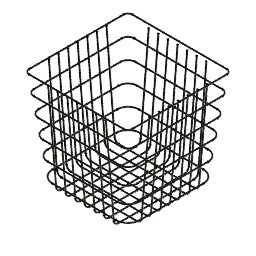
Living Roof Little Library Fusion Design File (Autodesk Fusion 360 archive; units mm, degrees)
design "Wire Basket"
Autodesk Fusion 360 part; units mm, degrees
note: some values were not read from the file. Chosen so that the rebuilt part matches the saved one: which bodies a step acts on.
sketch "Sketch1" plane through (0, 0, 0) normal (0, 1, 0) x (1, 0, 0)
  line L0 (0, 0) -> (104.7294, 0)
  line L1 (117.381, -11.5931) -> (139.7, -266.7)
  line L2 (0, -1.75) -> (0, -22.5)
  line L3 (1.75, 0) -> (22.5, 0)
  arc A0 (117.381, -11.5931) -> (104.7294, 0) centre (104.7294, -12.7) ccw
  line L4 (139.7, -266.7) -> (147.5, -266.7) construction
  circle A1 centre (143.7, -266.7) radius 2
  circle A2 centre (139.2902, -216.2955) radius 2
  circle A3 centre (134.8804, -165.891) radius 2
  circle A4 centre (130.4705, -115.4865) radius 2
  circle A5 centre (126.0607, -65.082) radius 2
  circle A6 centre (121.6509, -14.6776) radius 2
  dimension "d1" = 139.7
  dimension "d9" = 266.7
  dimension "d10" = 85
  dimension "d11" = 12.7
  dimension "d14" = 4
  dimension "d15" = 4
  dimension "d19" = 0
  constraint coincident L0.start origin
  constraint horizontal L0
  constraint tangent L0 A0
  constraint tangent L1 A0
  constraint horizontal L4
  constraint coincident L4 A1.centre
  measures "d1" distance of L1.end L2
  measures "d9" vertical distance of L0.start L1.end
  measures "d10" angle of L1 L3
  measures "d11" radius of A0
  measures "d14" diameter of A1
  measures "d15" distance of L1.end A1.centre
sketch "Sketch2" plane through (0, 0, 0) normal (1, 0, 0) x (0, 1, 0)
  circle A0 centre (0, 0) radius 2
  dimension "d12" = 4
  constraint coincident A0.centre origin
  measures "d12" diameter of A0
ref_plane "WorkPlane1" through (0, 0, 266.7) normal (0, 0, 1) x (1, 0, 0)
sweep "Sweep1" add profiles "Sketch2" path "Sketch1" along L0 A0 L1 section 1 makes body 1
sketch "Sketch3" plane through (0, 0, 266.7) normal (0, 0, 1) x (1, 0, 0)
  line L0 (0, 0) -> (0, -193.7) construction
  line L1 (143.7, 0) -> (143.7, -131)
  line L2 (131, -143.7) -> (0, -143.7)
  line L3 (0, 0) -> (143.7, -143.7) construction
  line L4 (135.0176, 0) -> (135.0176, -122.3176)
  line L5 (122.3176, -135.0176) -> (0, -135.0176)
  line L6 (126.3352, 0) -> (126.3352, -113.6352)
  line L7 (113.6352, -126.3352) -> (0, -126.3352)
  line L8 (117.6528, 0) -> (117.6528, -104.9528)
  line L9 (104.9528, -117.6528) -> (0, -117.6528)
  line L10 (108.9704, 0) -> (108.9704, -96.2704)
  line L11 (96.2704, -108.9704) -> (0, -108.9704)
  line L12 (100.288, 0) -> (100.288, -87.588)
  line L13 (87.588, -100.288) -> (0, -100.288)
  arc A0 (87.588, -100.288) -> (100.288, -87.588) centre (87.588, -87.588) ccw
  arc A1 (96.2704, -108.9704) -> (108.9704, -96.2704) centre (96.2704, -96.2704) ccw
  arc A2 (104.9528, -117.6528) -> (117.6528, -104.9528) centre (104.9528, -104.9528) ccw
  arc A3 (113.6352, -126.3352) -> (126.3352, -113.6352) centre (113.6352, -113.6352) ccw
  arc A4 (122.3176, -135.0176) -> (135.0176, -122.3176) centre (122.3176, -122.3176) ccw
  line L14 (0, 0) -> (147.5, 0) construction
  arc A5 (131, -143.7) -> (143.7, -131) centre (131, -131) ccw
  point P0 (143.7, 0)
  point P1 (139.2902, 0)
  point P2 (147.5, 0)
  dimension "d32" = 143.7
  dimension "d85" = 12.7
  dimension "d86" = 12.7
  dimension "d87" = 12.7
  dimension "d88" = 12.7
  dimension "d89" = 12.7
  dimension "d90" = 8.6824
  dimension "d91" = 8.6824
  dimension "d92" = 8.6824
  dimension "d93" = 8.6824
  dimension "d94" = 8.6824
  dimension "d95" = 12.7
  constraint coincident L0.start L3.start
  constraint vertical L0
  constraint coincident P0 L1.start
  constraint coincident L0 L2.end
  constraint perpendicular L0 L2
  constraint vertical L1
  constraint tangent L13 A0
  constraint tangent L12 A0
  constraint tangent L11 A1
  constraint tangent L10 A1
  constraint tangent L9 A2
  constraint tangent L8 A2
  constraint tangent L7 A3
  constraint tangent L6 A3
  constraint tangent L5 A4
  constraint tangent L4 A4
  constraint vertical L12
  constraint vertical L10
  constraint vertical L8
  constraint vertical L6
  constraint vertical L4
  constraint horizontal L5
  constraint horizontal L7
  constraint horizontal L9
  constraint horizontal L11
  constraint horizontal L13
  constraint coincident L3 A0.centre
  constraint coincident L3 A1.centre
  constraint coincident L3 A2.centre
  constraint coincident L3 A3.centre
  constraint coincident L3 A4.centre
  constraint coincident L0 L13.end
  constraint coincident L0 L11.end
  constraint coincident L0 L9.end
  constraint coincident L0 L7.end
  constraint coincident L0 L5.end
  constraint coincident P2 L14.end
  constraint coincident L14 L12.start
  constraint coincident L14 L10.start
  constraint coincident L14 L8.start
  constraint coincident L14 L6.start
  constraint coincident L14 L4.start
  constraint coincident L2 L3.end
  constraint coincident L1 L3.end
  constraint tangent L2 A5
  constraint tangent L1 A5
  measures "d32" distance of L0.start L2
  measures "d85" radius of A0
  measures "d86" radius of A1
  measures "d87" radius of A2
  measures "d88" radius of A3
  measures "d89" radius of A4
  measures "d90" distance of L2 L5
  measures "d91" distance of L5 L7
  measures "d92" distance of L7 L9
  measures "d93" distance of L9 L11
  measures "d94" distance of L11 L13
  measures "d95" radius of A5
sweep "Sweep2" add profiles "Sketch1" path "Sketch3" along L2 A5 L1 section 1 contours A1 separate body makes body 2
sweep "Sweep3" add profiles "Sketch1" path "Sketch3" along L12 A0 L13 section 1 contours A6 separate body makes body 3
sweep "Sweep4" add profiles "Sketch1" path "Sketch3" along L11 A1 L10 section 1 contours A5 separate body makes body 4
sweep "Sweep5" add profiles "Sketch1" path "Sketch3" along L9 A2 L8 section 1 contours A4 separate body makes body 5
sweep "Sweep6" add profiles "Sketch1" path "Sketch3" along L6 A3 L7 section 1 contours A3 separate body makes body 6
sweep "Sweep7" add profiles "Sketch1" path "Sketch3" along L5 A4 L4 section 1 contours A2 separate body makes body 7
pattern_linear "R-Pattern1" count 4 spacing 26.6667 along (0, -1, 0) of bodies 1 makes body 8 at (131.8461, -28.623, 181.7006) makes body 9 at (131.8461, -55.2896, 181.7006) makes body 10 at (131.8461, -81.9563, 181.7006)
mirror "Mirror1" about plane through (0, 0, 0) normal (1, 0, 0) of bodies 1 8 9 10 makes body 11 at (-131.8461, -1.9563, 181.7006) makes body 12 at (-131.8461, -28.623, 181.7006) makes body 13 at (-131.8461, -55.2896, 181.7006) makes body 14 at (-131.8461, -81.9563, 181.7006)
mirror "Mirror2" about plane through (0, 0, 0) normal (0, 1, 0) of bodies 14 12 13 8 9 10 makes body 15 at (131.8461, 28.623, 181.7006) makes body 16 at (131.8461, 55.2896, 181.7006) makes body 17 at (131.8461, 81.9563, 181.7006) makes body 18 at (-131.8461, 28.623, 181.7006) makes body 19 at (-131.8461, 55.2896, 181.7006) makes body 20 at (-131.8461, 81.9563, 181.7006)
mirror "Mirror3" about plane through (0, 0, 0) normal (1, 0, 0) of bodies 2 4 3 6 5 7 makes body 21 at (-145.6382, -43.6667, 267.1935) makes body 22 at (-120.5658, -29.196, 12.9975) makes body 23 at (-128.0508, -64.1802, 64.8829) makes body 24 at (-132.468, -69.9685, 115.3868) makes body 25 at (-136.8779, -75.7568, 165.9907) makes body 26 at (-141.2802, -40.7725, 216.4946)
mirror "Mirror4" about plane through (0, 0, 0) normal (0, 1, 0) of bodies 21 26 25 24 23 22 7 6 2 3 4 5 makes body 27 at (145.6382, 43.6667, 267.1935) makes body 28 at (120.5658, 29.196, 12.9975) makes body 29 at (128.0508, 64.1802, 64.8829) makes body 30 at (132.468, 69.9685, 115.3868) makes body 31 at (136.8779, 75.7568, 165.9907) makes body 32 at (141.2802, 40.7725, 216.4946) makes body 33 at (-145.6382, 43.6667, 267.1935) makes body 34 at (-120.5658, 29.196, 12.9975) makes body 35 at (-128.0508, 64.1802, 64.8829) makes body 36 at (-132.468, 69.9685, 115.3868) makes body 37 at (-136.8779, 75.7568, 165.9907) makes body 38 at (-141.2802, 40.7725, 216.4946)
copy_body "CopyPasteBodies1" bodies 12 13 14 15 16 17 18 19 20 11 10 9 8 1 makes body 39 makes body 40 makes body 41 makes body 42 makes body 43 makes body 44 makes body 45 makes body 46 makes body 47 makes body 48 makes body 49 makes body 50 makes body 51 makes body 52
move_body "Move2" bodies 39 40 41 42 43 44 45 46 47 48 49 50 51 52 to x (0, 1, 0) y (-1, 0, 0) z (0, 0, 1) at (0, -2, -4)
ref_plane "WorkPlane2" through (0, 0, 268.7) normal (0, 0, 1) x (1, 0, 0)
equation "d1 = basketWidth / 2"
equation "basketWidth = 11 in" comment "Width of Basket"
equation "basketHeight = 10.5 in" comment "Height of Basket"
equation "numVert = 6" comment "Number of vertical wires"
equation "numHoriz = 5" comment "Number of horizontal bars"
equation "wireDia = 4 mm" comment "Diameter of wire"
equation "bendRad = 0.5 in" comment "Radius of bends"
equation "edgeSlope = 85 deg" comment "Angle the basket flares out"
equation "d9 = basketHeight"
equation "d10 = edgeSlope"
equation "d11 = bendRad"
equation "d12 = wireDia"
equation "d14 = wireDia"
equation "d15 = wireDia"
equation "d16 = numVert"
equation "d18 = -( basketHeight * sin(edgeSlope) - bendRad )"
equation "d20 = basketHeight"
equation "d32 = basketWidth / 2 + wireDia"
equation "d85 = bendRad"
equation "d86 = bendRad"
equation "d87 = bendRad"
equation "d88 = bendRad"
equation "d89 = bendRad"
equation "d91 = d90"
equation "d92 = d90"
equation "d93 = d90"
equation "d94 = d90"
equation "d95 = bendRad"
equation "d100 = basketHeight + ( wireDia / 2 )"
